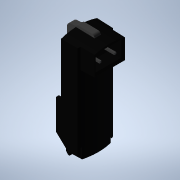
# Autodesk Inventor part: 566714 VAVE-L1-1VH2-LP
Saved by Autodesk Inventor 2021 (Build 250183000, 183)
## iProperties
Created: 2026-04-16
Part Number: 566714 VAVE-L1-1VH2-LP
Material: Generic
Catalog Web Link: www.3dfindit.com
Description: VAVE-Electrical connecting components
Vendor: FESTO
Document SubType Name: Modeling
Designer: psAdmin
Manufacturer: FESTO
Mass: 1.5 g
Surface Area: 13.2974 cm^2
Volume: 1.29606 cm^3
Density: 1 g/cm^3
Appearance: PSOLRGB-80-80-80
Category: PARTsolutions
Company: FESTO
Title: 566714 VAVE-L1-1VH2-LP
Author: Cadenas PARTsolutions
Comments: Electrical connecting components
PSOL_IDENT_0: {$CADENAS_DATA/23d-libs/festo/parts/v/vave/vave.prj},182 {VTYP=3D},{NB=566714 VAVE-L1-1VH2-LP},{LINA=
PSOL_IDENT_1: 566714 VAVE-L1-1VH2-LP},{NN=VAVE},{DATE=14.11.2025 15:28:53},{GEOMDATE=14.11.2025 15:28:00},{VERSION=
PSOL_IDENT_2: },{LINEID=10},{WBVAR=},{WBNUMERIC=}  {NB=566714 VAVE-L1-1VH2-LP},{LINA=566714 VAVE-L1-1VH2-LP},{KT=D
PSOL_IDENT_3: UMMY},{TNR=566714},{TYP=VAVE-L1-1VH2-LP},{VERS=H2},{H100=23.512},{L100=0},{VERS2=1},{CNSMASSEXACT=0.
PSOL_IDENT_4: 0015},{GTIN=4052568057541}
NB: 566714 VAVE-L1-1VH2-LP
NN: VAVE
NT: Electrical connecting components
NBSYN: $TNR. $TYP.
LINA: 566714 VAVE-L1-1VH2-LP
CATALOG: Festo
TNR: 566714
TYP: VAVE-L1-1VH2-LP
CNSMASSEXACT: 0.0015
GTIN: 4052568057541
SUPPLIER: FESTO
ARTICLENO: 566714 VAVE-L1-1VH2-LP
BOMINFO: 566714 VAVE-L1-1VH2-LP
CREATOR: CADENAS GmbH
Autodesk Inventor part; units mm, degrees
sketch "Sketch_23" plane through (0, 0, 0) normal (0, 0, 1) x (1, 0, 0)
  line L0 (-6.5, 14.7231) -> (-6.5, 4.0058)
  line L1 (-6.5, 4.0058) -> (-3.404, 0.9098)
  line L2 (-3.404, 0.9098) -> (-2.55, 0.8949)
  line L3 (-2.55, 0.8949) -> (-2.55, 0.5951)
  line L4 (-2.55, 0.5951) -> (-4.4413, 0.5621)
  arc A0 (-4.4413, 0.5621) -> (-4.8099, -0.2659) centre (-4.4326, 0.0622) ccw
  line L5 (-4.8099, -0.2659) -> (-4.3557, -0.7885)
  arc A1 (-4.3557, -0.7885) -> (-4.1395, -0.8847) centre (-4.1443, -0.6048) ccw
  line L6 (-4.1395, -0.8847) -> (-3.9988, -0.8823)
  arc A2 (-3.9988, -0.8823) -> (-3.9044, -0.7547) centre (-4.0006, -0.7823) ccw
  line L7 (-3.9044, -0.7547) -> (-4.0447, -0.2655)
  arc A3 (-3.9521, -0.138) -> (-4.0447, -0.2655) centre (-3.9486, -0.2379) ccw
  line L8 (-3.9521, -0.138) -> (0, 0)
  line L9 (0, 0) -> (0, 29)
  line L10 (0, 29) -> (-5.2, 29)
  line L11 (-5.2, 29) -> (-5.2, 15.3866)
  arc A4 (-5.4739, 15.0878) -> (-5.2, 15.3866) centre (-5.5, 15.3866) ccw
  line L12 (-5.4739, 15.0878) -> (-6.2261, 15.022)
  arc A5 (-6.2261, 15.022) -> (-6.5, 14.7231) centre (-6.2, 14.7231) ccw
  constraints: 26 end point, 12 point on circle, 6 centre point
extrude "Extrusion1" add sketch "Sketch_23" along normal mid plane 10
sketch "Sketch_1" plane through (0, -5, 0) normal (0, 1, 0) x (1, 0, 0)
  line L0 (-7, -10) -> (5, -10)
  line L1 (5, -10) -> (5, 10)
  line L2 (5, 10) -> (-7, 10)
  line L3 (-7, 10) -> (-7, -10)
  line L4 (-6.5, -4.934) -> (-0.7835, -4.7843)
  arc A0 (-0.7835, -4.7843) -> (-0.7835, 4.7843) centre (-15, 0) ccw
  line L5 (-0.7835, 4.7843) -> (-6.5, 4.934)
  line L6 (-6.5, 4.934) -> (-6.5, -4.934)
  constraints: 14 end point, 2 point on circle, 1 centre point
sketch "Sketch_3" plane through (0, 0, 0) normal (1, 0, 0) x (0, 1, 0)
  line L0 (1.164, 5) -> (-3, 5)
  line L1 (-3, 5) -> (-3, -5)
  line L2 (-3, -5) -> (1.164, -5)
  line L3 (1.164, -5) -> (1.164, -4.23)
  line L4 (1.164, -4.23) -> (2.722, -4.23)
  arc A0 (2.722, -4.23) -> (2.722, -3.851) centre (2.722, -4.0405) ccw
  line L5 (2.722, -3.851) -> (-1, -3.851)
  line L6 (-1, -3.851) -> (-1, -2.1245)
  line L7 (-1, -2.1245) -> (-0.9, -2.1245)
  line L8 (-0.9, -2.1245) -> (-0.9, 2.1245)
  line L9 (-0.9, 2.1245) -> (-1, 2.1245)
  line L10 (-1, 2.1245) -> (-1, 3.851)
  line L11 (-1, 3.851) -> (2.722, 3.851)
  arc A1 (2.722, 3.851) -> (2.722, 4.23) centre (2.722, 4.0405) ccw
  line L12 (2.722, 4.23) -> (1.164, 4.23)
  line L13 (1.164, 4.23) -> (1.164, 5)
  constraints: 28 end point, 4 point on circle, 2 centre point
sketch "Sketch_4" plane through (0, 0, 0) normal (0, 1, 0) x (-1, 0, 0)
  line L0 (6.4, 2.2572) -> (3.6843, 2.1149)
  arc A0 (3.6843, 2.1149) -> (3.4, 1.8153) centre (3.7, 1.8153) ccw
  line L1 (3.4, 1.8153) -> (3.4, -1.8153)
  arc A1 (3.4, -1.8153) -> (3.6843, -2.1149) centre (3.7, -1.8153) ccw
  line L2 (3.6843, -2.1149) -> (6.4, -2.2572)
  line L3 (6.4, -2.2572) -> (6.4, 2.2572)
  constraints: 8 end point, 4 point on circle, 2 centre point
extrude "Extrusion2" cut sketch "Sketch_4" along normal mid plane 2
sketch "Sketch_5" plane through (0, 0, 0) normal (0, 0, 1) x (1, 0, 0)
  line L0 (-15, 0.1264) -> (-15, 3.912)
  line L1 (-15, 3.912) -> (-0.55, 3.912)
  line L2 (-0.55, 3.912) -> (-0.55, 0.9207)
  arc A0 (-0.8395, 0.6209) -> (-0.55, 0.9207) centre (-0.85, 0.9207) ccw
  line L3 (-0.8395, 0.6209) -> (-15, 0.1264)
  line L4 (-15, 0.1264) -> (-15, 3.912)
  constraints: 10 end point, 2 point on circle, 1 centre point
revolve "Revolution1" cut sketch "Sketch_5" angle 60 mid plane about axis through (-15, 0.1264, 0) along (0, 1, 0)
sketch "Sketch_6" plane through (0, 0, 5) normal (0, 0, 1) x (1, 0, 0)
  line L0 (-6.5, 14.7231) -> (-6.5, 4.0058)
  line L1 (-6.5, 4.0058) -> (-3.404, 0.9098)
  line L2 (-3.404, 0.9098) -> (0, 0.8504)
  line L3 (0, 0.8504) -> (0, 27.33)
  line L4 (0, 27.33) -> (-5.2, 27.33)
  line L5 (-5.2, 27.33) -> (-5.2, 15.3866)
  arc A0 (-5.4739, 15.0878) -> (-5.2, 15.3866) centre (-5.5, 15.3866) ccw
  line L6 (-5.4739, 15.0878) -> (-6.2261, 15.022)
  arc A1 (-6.2261, 15.022) -> (-6.5, 14.7231) centre (-6.2, 14.7231) ccw
  constraints: 14 end point, 4 point on circle, 2 centre point
sketch "Sketch_7" plane through (0, 0, -5) normal (0, 0, 1) x (1, 0, 0)
  line L0 (-6.5, 14.7231) -> (-6.5, 4.0058)
  line L1 (-6.5, 4.0058) -> (-3.404, 0.9098)
  line L2 (-3.404, 0.9098) -> (0, 0.8504)
  line L3 (0, 0.8504) -> (0, 27.33)
  line L4 (0, 27.33) -> (-5.2, 27.33)
  line L5 (-5.2, 27.33) -> (-5.2, 15.3866)
  arc A0 (-5.4739, 15.0878) -> (-5.2, 15.3866) centre (-5.5, 15.3866) ccw
  line L6 (-5.4739, 15.0878) -> (-6.2261, 15.022)
  arc A1 (-6.2261, 15.022) -> (-6.5, 14.7231) centre (-6.2, 14.7231) ccw
  constraints: 14 end point, 4 point on circle, 2 centre point
extrude "Extrusion3" cut sketch "Sketch_3" against normal blind 7
extrude "Extrusion4" add sketch "Sketch_6" against normal blind 0.77
extrude "Extrusion5" add sketch "Sketch_7" along normal blind 0.77
sketch "Sketch_12" plane through (0, 0.85, 0) normal (0, 1, 0) x (1, 0, 0)
  line L0 (-6.5, -4.384) -> (-1.2087, -4.2454)
  arc A0 (-1.2087, -4.2454) -> (-1.2087, 4.2454) centre (-15, 0) ccw
  line L1 (-1.2087, 4.2454) -> (-6.5, 4.384)
  line L2 (-6.5, 4.384) -> (-6.5, -4.384)
  constraints: 6 end point, 2 point on circle, 1 centre point
extrude "Extrusion6" cut sketch "Sketch_12" along normal blind 3.062
sketch "Sketch_8" plane through (0, 0, 0) normal (0, 0, 1) x (1, 0, 0)
  line L0 (-3.603, 3.7107) -> (-3.603, 3.5593)
  arc A0 (-3.603, 3.5593) -> (-3.4556, 3.4093) centre (-3.453, 3.5593) ccw
  line L1 (-3.4556, 3.4093) -> (0, 3.349)
  line L2 (0, 3.349) -> (0, 3.921)
  line L3 (0, 3.921) -> (-3.4556, 3.8607)
  arc A1 (-3.4556, 3.8607) -> (-3.603, 3.7107) centre (-3.453, 3.7107) ccw
  constraints: 8 end point, 4 point on circle, 2 centre point
extrude "Extrusion7" add sketch "Sketch_8" along normal mid plane 10
sketch "Sketch_9" plane through (0, 0, -2.693) normal (0, 0, 1) x (1, 0, 0)
  line L0 (-4.154, 0.508) -> (0, 0.508)
  line L1 (0, 0.508) -> (0, 3.405)
  line L2 (0, 3.405) -> (-1.604, 3.405)
  line L3 (-1.604, 3.405) -> (-1.604, 1.1255)
  arc A0 (-1.7693, 0.9285) -> (-1.604, 1.1255) centre (-1.804, 1.1255) ccw
  line L4 (-1.7693, 0.9285) -> (-4.154, 0.508)
  constraints: 10 end point, 2 point on circle, 1 centre point
extrude "Extrusion8" add sketch "Sketch_9" against normal blind 0.512
sketch "Sketch_10" plane through (0, 0, 2.693) normal (0, 0, 1) x (1, 0, 0)
  line L0 (-4.154, 0.508) -> (0, 0.508)
  line L1 (0, 0.508) -> (0, 3.405)
  line L2 (0, 3.405) -> (-1.604, 3.405)
  line L3 (-1.604, 3.405) -> (-1.604, 1.1255)
  arc A0 (-1.7693, 0.9285) -> (-1.604, 1.1255) centre (-1.804, 1.1255) ccw
  line L4 (-1.7693, 0.9285) -> (-4.154, 0.508)
  constraints: 10 end point, 2 point on circle, 1 centre point
extrude "Extrusion9" add sketch "Sketch_10" along normal blind 0.512
sketch "Sketch_15" plane through (0, 2, 0) normal (0, 1, 0) x (1, 0, 0)
  line L0 (-6.5, -4.384) -> (-5.2, -4.35)
  line L1 (-5.2, -4.35) -> (-5.2, 4.35)
  line L2 (-5.2, 4.35) -> (-6.5, 4.384)
  line L3 (-6.5, 4.384) -> (-6.5, -4.384)
  constraints: 8 end point
extrude "Extrusion10" cut sketch "Sketch_15" along normal blind 30
sketch "Sketch_13" plane through (0, 0, 0) normal (0, 0, 1) x (1, 0, 0)
  line L0 (-8.2, 10.398) -> (-6.5, 10.398)
  line L1 (-6.5, 10.398) -> (-6.5, 12.1231)
  arc A0 (-6.2261, 12.422) -> (-6.5, 12.1231) centre (-6.2, 12.1231) ccw
  line L2 (-6.2261, 12.422) -> (-5.3826, 12.4958)
  arc A1 (-5.3826, 12.4958) -> (-5.2, 12.695) centre (-5.4, 12.695) ccw
  line L3 (-5.2, 12.695) -> (-5.2, 30.398)
  line L4 (-5.2, 30.398) -> (-8.2, 30.398)
  line L5 (-8.2, 30.398) -> (-8.2, 10.398)
  constraints: 12 end point, 4 point on circle, 2 centre point
extrude "Extrusion11" cut sketch "Sketch_13" along normal blind 5
extrude "Extrusion12" cut sketch "Sketch_1" along normal blind 35
sketch "Sketch_14" plane through (-5.5, 0, 0) normal (1, 0, 0) x (0, 0, -1)
  line L0 (-4.25, 29.912) -> (-4.25, 3.912)
  line L1 (-4.25, 3.912) -> (4.25, 3.912)
  line L2 (4.25, 3.912) -> (4.25, 29.912)
  line L3 (4.25, 29.912) -> (-4.25, 29.912)
  constraints: 8 end point
extrude "Extrusion13" add sketch "Sketch_14" along normal blind 1.5
sketch "Sketch_17" plane through (-5.5, 0, 0) normal (1, 0, 0) x (0, 0, -1)
  line L0 (-4.25, 30.812) -> (-4.25, 25.812)
  line L1 (-4.25, 25.812) -> (4.25, 25.812)
  line L2 (4.25, 25.812) -> (4.25, 30.812)
  line L3 (4.25, 30.812) -> (-4.25, 30.812)
  constraints: 8 end point
extrude "Extrusion14" cut sketch "Sketch_17" along normal blind 0.3
sketch "Sketch_11" plane through (3.15, 0, 0) normal (1, 0, 0) x (0, 0, -1)
  line L0 (-4.144, 27.593) -> (-4.144, 21.162)
  line L1 (-4.144, 21.162) -> (4.144, 21.162)
  line L2 (4.144, 21.162) -> (4.144, 27.593)
  line L3 (4.144, 27.593) -> (-4.144, 27.593)
  constraints: 8 end point
extrude "Extrusion15" add sketch "Sketch_11" against normal blind 6 draft 1
sketch "Sketch_16" plane through (0, 0, 0) normal (0, 0, 1) x (1, 0, 0)
  line L0 (3.3, 12.312) -> (-5.2, 12.312)
  line L1 (-5.2, 32.312) -> (-5.2, 27.312)
  line L2 (-5.2, 27.312) -> (3.3, 27.0894)
  line L3 (3.3, 27.0894) -> (3.3, 32.312)
  line L4 (3.3, 32.312) -> (-5.2, 32.312)
  constraints: 10 end point
revolve "Revolution2" cut sketch "Sketch_16" angle 40 mid plane about axis through (3.3, 12.312, 0) along (-1, 0, 0)
sketch "Sketch_19" plane through (2.78, 0, 0) normal (1, 0, 0) x (0, 0, -1)
  line L0 (-3.483, 26.19) -> (-3.483, 21.83)
  line L1 (-3.483, 21.83) -> (3.477, 21.83)
  line L2 (3.477, 21.83) -> (3.477, 26.19)
  line L3 (3.477, 26.19) -> (-3.483, 26.19)
  constraints: 8 end point
extrude "Extrusion16" cut sketch "Sketch_19" along normal blind 2 draft 45
sketch "Sketch_20" plane through (2.78, 0, 0) normal (1, 0, 0) x (0, 0, -1)
  line L0 (-3.483, 26.19) -> (-3.483, 21.83)
  line L1 (-3.483, 21.83) -> (3.477, 21.83)
  line L2 (3.477, 21.83) -> (3.477, 26.19)
  line L3 (3.477, 26.19) -> (-3.483, 26.19)
  constraints: 8 end point
extrude "Extrusion17" cut sketch "Sketch_20" against normal blind 3.38
sketch "Sketch_21" plane through (-0.604, 0, 0) normal (1, 0, 0) x (0, 0, -1)
  line L0 (1.75, 23.762) -> (1.75, 23.262)
  line L1 (1.75, 23.262) -> (2.25, 23.262)
  line L2 (2.25, 23.262) -> (2.25, 23.762)
  line L3 (2.25, 23.762) -> (1.75, 23.762)
  constraints: 8 end point
extrude "Extrusion18" add sketch "Sketch_21" along normal blind 3.25
sketch "Sketch_22" plane through (-0.604, 0, 0) normal (1, 0, 0) x (0, 0, -1)
  line L0 (-2.25, 23.762) -> (-2.25, 23.262)
  line L1 (-2.25, 23.262) -> (-1.75, 23.262)
  line L2 (-1.75, 23.262) -> (-1.75, 23.762)
  line L3 (-1.75, 23.762) -> (-2.25, 23.762)
  constraints: 8 end point
extrude "Extrusion19" add sketch "Sketch_22" along normal blind 3.25
sketch "Sketch_27" plane through (0, 0, 0) normal (0, 0, 1) x (1, 0, 0)
  line L0 (-0.62, 25.39) -> (1.98, 25.39)
  line L1 (1.98, 25.39) -> (2.78, 26.19)
  line L2 (2.78, 26.19) -> (-0.62, 26.19)
  line L3 (-0.62, 26.19) -> (-0.62, 25.39)
  constraints: 8 end point
extrude "Extrusion20" add sketch "Sketch_27" along normal mid plane 2.25
sketch "Sketch_29" plane through (0, 0, 0) normal (0, 0, 1) x (1, 0, 0)
  line L0 (-0.6, 25.39) -> (2.78, 25.39)
  line L1 (2.78, 25.39) -> (2.78, 26.19)
  line L2 (2.78, 26.19) -> (-0.6, 26.19)
  line L3 (-0.6, 26.19) -> (-0.6, 25.39)
  constraints: 8 end point
extrude "Extrusion21" cut sketch "Sketch_29" along normal mid plane 1.5
sketch "Sketch_45" plane through (0, 21.104, 0) normal (0, 1, 0) x (1, 0, 0)
  line L0 (-1.1, 1.5) -> (-1.1, -1.5)
  line L1 (-1.1, -1.5) -> (1.2, -1.5)
  arc A0 (1.2, -1.5) -> (1.4, -1.3) centre (1.2, -1.3) ccw
  line L2 (1.4, -1.3) -> (1.4, 1.3)
  arc A1 (1.4, 1.3) -> (1.2, 1.5) centre (1.2, 1.3) ccw
  line L3 (1.2, 1.5) -> (-1.1, 1.5)
  constraints: 8 end point, 4 point on circle, 2 centre point
extrude "Extrusion22" cut sketch "Sketch_45" along normal mid plane 1
sketch "Sketch_2" plane through (-5.5, 0, 0) normal (1, 0, 0) x (0, 0, -1)
  line L0 (1.0745, 5.255) -> (1.9255, 5.255)
  line L1 (1.9255, 5.255) -> (1.9255, 9.106)
  line L2 (1.9255, 9.106) -> (1.0745, 9.106)
  line L3 (1.0745, 9.106) -> (1.0745, 5.255)
  constraints: 8 end point
extrude "Extrusion23" cut sketch "Sketch_2" along normal blind 1.05 draft -1
sketch "Sketch_24" plane through (-5.5, 0, 0) normal (1, 0, 0) x (0, 0, -1)
  line L0 (-1.9255, 5.255) -> (-1.0745, 5.255)
  line L1 (-1.0745, 5.255) -> (-1.0745, 9.106)
  line L2 (-1.0745, 9.106) -> (-1.9255, 9.106)
  line L3 (-1.9255, 9.106) -> (-1.9255, 5.255)
  constraints: 8 end point
extrude "Extrusion24" cut sketch "Sketch_24" along normal blind 1.05 draft -1
sketch "Sketch_25" plane through (0, 0, -1.5) normal (0, 0, 1) x (1, 0, 0)
  line L0 (-3.45, 7.162) -> (-5.5, 7.162)
  line L1 (-5.5, 7.162) -> (-5.5, 8.012)
  line L2 (-5.5, 8.012) -> (-3.45, 7.9404)
  line L3 (-3.45, 7.9404) -> (-3.45, 7.162)
  line L4 (-3.45, 7.162) -> (-5.5, 7.162)
  constraints: 10 end point
revolve "Revolution3" cut sketch "Sketch_25" angle 360 about axis through (-3.45, 7.162, -1.5) along (1, 0, 0)
sketch "Sketch_26" plane through (0, 0, 1.5) normal (0, 0, 1) x (1, 0, 0)
  line L0 (-3.45, 7.162) -> (-5.5, 7.162)
  line L1 (-5.5, 7.162) -> (-5.5, 8.012)
  line L2 (-5.5, 8.012) -> (-3.45, 7.9404)
  line L3 (-3.45, 7.9404) -> (-3.45, 7.162)
  line L4 (-3.45, 7.162) -> (-5.5, 7.162)
  constraints: 10 end point
revolve "Revolution4" cut sketch "Sketch_26" angle 360 about axis through (-3.45, 7.162, 1.5) along (1, 0, 0)
sketch "Sketch_40" plane through (0, 0, 0) normal (0, 0, 1) x (1, 0, 0)
  line L0 (-7.6, 26.3683) -> (-7.6, 22.574)
  line L1 (-7.6, 22.574) -> (-2.1, 17.959)
  line L2 (-2.1, 17.959) -> (-2.1, 26.5)
  line L3 (-2.1, 26.5) -> (-0.1, 26.5)
  line L4 (-0.1, 26.5) -> (-0.1, 27.0465)
  arc A0 (-0.1, 27.0465) -> (-0.886, 27.8464) centre (-0.9, 27.0465) ccw
  line L5 (-0.886, 27.8464) -> (-4.704, 27.913)
  line L6 (-4.704, 27.913) -> (-5.5, 27.4073)
  line L7 (-5.5, 27.4073) -> (-6.6349, 27.3677)
  arc A1 (-6.6349, 27.3677) -> (-7.6, 26.3683) centre (-6.6, 26.3683) ccw
  constraints: 16 end point, 4 point on circle, 2 centre point
extrude "Extrusion25" add sketch "Sketch_40" along normal mid plane 1.722
ref_plane "MHA1_XY" through (-5.5, 19, 0) normal (1, 0, 0) x (0, 0, -1)
ref_plane "MHA1_YZ" through (-5.5, 19, 0) normal (0, 0, -1) x (0, 1, 0)
ref_plane "MHA1_ZX" through (-5.5, 19, 0) normal (0, 1, 0) x (1, 0, 0)
ref_plane "NEBV_XY" through (-0.004, 23.512, 0) normal (1, 0, 0) x (0, 0, -1)
ref_plane "NEBV_YZ" through (-0.004, 23.512, 0) normal (0, 0, -1) x (0, 1, 0)
ref_plane "NEBV_ZX" through (-0.004, 23.512, 0) normal (0, 1, 0) x (1, 0, 0)
ref_plane "VAVE_XY" through (-4.28, 0, 0) normal (0, -1, 0) x (1, 0, 0)
ref_plane "VAVE_YZ" through (-4.28, 0, 0) normal (1, 0, 0) x (0, 0, 1)
ref_plane "VAVE_ZX" through (-4.28, 0, 0) normal (0, 0, 1) x (0, -1, 0)
body "Solid1"
